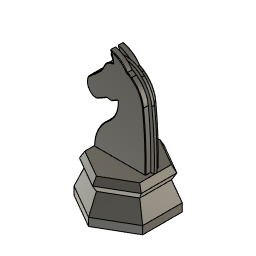
Knight Chess Piece (Autodesk Fusion 360 design; units mm, degrees)
Autodesk Fusion 360 part; units mm, degrees
sketch "Sketch2" plane through (0, 0, 0) normal (0, 0, 1) x (1, 0, 0)
  line L0 (0, 15) -> (-12.990381, 7.5)
  line L1 (-12.990381, 7.5) -> (-12.990381, -7.5)
  line L2 (-12.990381, -7.5) -> (0, -15)
  line L3 (0, -15) -> (12.990381, -7.5)
  line L4 (12.990381, -7.5) -> (12.990381, 7.5)
  line L5 (12.990381, 7.5) -> (0, 15)
  dimension "d4" = 15
  measures "d4" distance of L0.start origin
extrude "Extrude1" add sketch "Sketch2" along normal blind 3 contours L0 L1 L2 L3 L4 L5 picked at (4.330127, 2.5)
sketch "Sketch3" plane through (0, 0, 3) normal (0, 0, 1) x (-1, 0, 0)
  line L0 (-12.990381, -7.5) -> (0, -15)
  line L1 (0, -15) -> (12.990381, -7.5)
  line L2 (12.990381, -7.5) -> (12.990381, 7.5)
  line L3 (12.990381, 7.5) -> (0, 15)
  line L4 (0, 15) -> (-12.990381, 7.5)
  line L5 (-12.990381, 7.5) -> (-12.990381, -7.5)
  line L6 (0, -15) -> (12.990381, -7.5)
  line L7 (12.990381, -7.5) -> (12.990381, 7.5)
  line L8 (12.990381, 7.5) -> (0, 15)
  line L9 (0, 15) -> (-12.990381, 7.5)
  line L10 (-12.990381, 7.5) -> (-12.990381, -7.5)
  line L11 (-12.990381, -7.5) -> (0, -15)
  constraint coincident L0.end L1.start
ref_plane "WorkPlane1" through (0, 0, 10) normal (0, 0, 1) x (-1, 0, 0)
sketch "Sketch4" plane through (0, 0, 10) normal (0, 0, 1) x (1, 0, 0)
  line L0 (0, 12) -> (-10.392305, 6)
  line L1 (-10.392305, 6) -> (-10.392305, -6)
  line L2 (-10.392305, -6) -> (0, -12)
  line L3 (0, -12) -> (10.392305, -6)
  line L4 (10.392305, -6) -> (10.392305, 6)
  line L5 (10.392305, 6) -> (0, 12)
  dimension "d8" = 12
  measures "d8" distance of L0.start origin
loft "Loft1" add profiles "Sketch3", "Sketch4" section 1 contours L0 L1 L2 L3 L4 L5 L6 L7 L8 L9 L10 L11 picked at (-4.330127, -2.5) section 2 contours L0 L1 L2 L3 L4 L5 picked at (0, 0)
sketch "Sketch5" plane through (0, 0, 10) normal (0, 0, 1) x (-1, 0, 0)
  line L0 (-10.392305, -6) -> (0, -12)
  line L1 (0, -12) -> (10.392305, -6)
  line L2 (10.392305, -6) -> (10.392305, 6)
  line L3 (10.392305, 6) -> (0, 12)
  line L4 (0, 12) -> (-10.392305, 6)
  line L5 (-10.392305, 6) -> (-10.392305, -6)
  line L6 (0, -12) -> (10.392305, -6)
  line L7 (10.392305, -6) -> (10.392305, 6)
  line L8 (10.392305, 6) -> (0, 12)
  line L9 (0, 12) -> (-10.392305, 6)
  line L10 (-10.392305, 6) -> (-10.392305, -6)
  line L11 (-10.392305, -6) -> (0, -12)
  constraint coincident L0.end L1.start
ref_plane "WorkPlane2" through (0, 0, 12.5) normal (0, 0, 1) x (-1, 0, 0)
sketch "Sketch6" plane through (0, 0, 12.5) normal (0, 0, 1) x (1, 0, 0)
  line L0 (0, 13.5) -> (-11.691343, 6.75)
  line L1 (-11.691343, 6.75) -> (-11.691343, -6.75)
  line L2 (-11.691343, -6.75) -> (0, -13.5)
  line L3 (0, -13.5) -> (11.691343, -6.75)
  line L4 (11.691343, -6.75) -> (11.691343, 6.75)
  line L5 (11.691343, 6.75) -> (0, 13.5)
  line L6 (0, 15) -> (0, 12)
  constraint midpoint L0.start L6
ref_plane "WorkPlane3" through (0, 0, 15) normal (0, 0, 1) x (1, 0, 0)
sketch "Sketch7" plane through (0, 0, 15) normal (0, 0, 1) x (1, 0, 0)
  line L0 (0, 12) -> (-10.392305, 6)
  line L1 (-10.392305, 6) -> (-10.392305, -6)
  line L2 (-10.392305, -6) -> (0, -12)
  line L3 (0, -12) -> (10.392305, -6)
  line L4 (10.392305, -6) -> (10.392305, 6)
  line L5 (10.392305, 6) -> (0, 12)
  point P0 (0, 12)
  constraint coincident P0 L0.start
loft "Loft2" add profiles "Sketch5", "Sketch6" section 1 contours L0 L1 L2 L3 L4 L5 L6 L7 L8 L9 L10 L11 picked at (-3.464102, 2) section 2 contours L0 L1 L2 L3 L4 L5 picked at (3.897114, 2.25)
sketch "Sketch8" plane through (0, 0, 12.5) normal (0, 0, 1) x (-1, 0, 0)
  line L0 (-11.691343, -6.75) -> (0, -13.5)
  line L1 (0, -13.5) -> (11.691343, -6.75)
  line L2 (11.691343, -6.75) -> (11.691343, 6.75)
  line L3 (11.691343, 6.75) -> (0, 13.5)
  line L4 (0, 13.5) -> (-11.691343, 6.75)
  line L5 (-11.691343, 6.75) -> (-11.691343, -6.75)
  line L6 (0, -13.5) -> (11.691343, -6.75)
  line L7 (11.691343, -6.75) -> (11.691343, 6.75)
  line L8 (11.691343, 6.75) -> (0, 13.5)
  line L9 (0, 13.5) -> (-11.691343, 6.75)
  line L10 (-11.691343, 6.75) -> (-11.691343, -6.75)
  line L11 (-11.691343, -6.75) -> (0, -13.5)
  constraint coincident L0.end L1.start
loft "Loft3" add profiles "Sketch8", "Sketch7" section 1 contours L0 L1 L2 L3 L4 L5 L6 L7 L8 L9 L10 L11 picked at (-3.897114, -2.25) section 2 contours L0 L1 L2 L3 L4 L5 picked at (0, 0)
shell "Shell1" thickness 2 removed faces 1 at (4.330127, 2.5, 0)
sketch "Sketch10" plane through (0, 0, 0) normal (0, 1, 0) x (1, 0, 0)
  line L0 (-15, 0) -> (15, 0) construction
  line L1 (15, 0) -> (15, -50) construction
  line L2 (15, -50) -> (-15, -50) construction
  line L3 (-15, -50) -> (-15, 0) construction
  line L4 (0, 0) -> (0, -50.000001) construction
  arc A0 (-10.392305, -15) -> (-5.031411, -25.974647) centre (4.068204, -14.733001) ccw
  arc A1 (-1.45223, -34.282944) -> (-5.031411, -25.974647) centre (-11.152568, -33.536714) ccw
  line L5 (-1.45223, -34.282944) -> (-3.369432, -33.194671)
  arc A2 (-3.369432, -33.194671) -> (-5.5, -33.194671) centre (-4.434716, -35.071372) ccw
  line L6 (-5.5, -33.194671) -> (-9.003186, -31.206135)
  arc A3 (-9.003186, -31.206135) -> (-11, -31.206135) centre (-10.001593, -32.965019) ccw
  arc A4 (-11, -31.206135) -> (-12.660134, -36.669443) centre (-8.953188, -34.811985) ccw
  line L7 (-12.660134, -36.669443) -> (-8.504363, -40.327582)
  arc A5 (-6.723878, -42.918601) -> (-8.504363, -40.327582) centre (-12.7535, -45.154747) ccw
  arc A6 (-4.682649, -45.182039) -> (3.634445, -44.218793) centre (-1.386515, -37.253958) ccw
  arc A7 (3.634445, -44.218793) -> (8.13983, -36.485073) centre (-2.802633, -35.289588) ccw
  line L8 (10.392305, -15) -> (0, -15)
  arc A8 (8.13983, -36.485073) -> (9.030382, -15) centre (-150.571914, -19.145511) ccw
  line L9 (-10.392305, -15) -> (9.030382, -15)
  arc A9 (-6.723878, -42.918601) -> (-4.682649, -45.182039) centre (-2.858972, -41.485262) ccw
  point P0 (-10.392305, -15)
  dimension "d13" = 30
  dimension "d14" = 50
  dimension "d15" = 15
  constraint horizontal L0
  constraint vertical L1
  constraint horizontal L2
  constraint coincident L4.start origin
  constraint perpendicular L2 L4
  constraint tangent A0 A1
  constraint tangent L5 A2
  constraint parallel L5 L6
  constraint tangent L6 A3
  constraint tangent A3 A4
  constraint tangent L7 A5
  constraint tangent A6 A7
  constraint tangent A7 A8
  constraint tangent A5 A9
  measures "d13" distance of L0.start L0.end
  measures "d14" distance of L0.start L2.end
  measures "d15" distance of L3 L4
extrude "Extrude2" add sketch "Sketch10" along normal mid plane 5 contours A0 A1 L5 A2 L6 A3 A4 L7 A5 A6 A7 L8 A8 L9 A9 picked at (1.669067, -21.354104)
sketch "Sketch12" plane through (0, 0, 0) normal (0, 1, 0) x (1, 0, 0)
  line L0 (-10.392305, -15) -> (8.638266, -15.045559)
  line L1 (-12.660134, -36.669443) -> (-8.504363, -40.327582)
  arc A0 (-11, -31.206135) -> (-12.660134, -36.669443) centre (-8.953188, -34.811985) ccw
  arc A1 (-5.268961, -44.810581) -> (4.41457, -43.289947) centre (-1.520828, -37.085915) ccw
  arc A2 (-7.025416, -42.576626) -> (-8.504363, -40.327582) centre (-11.871086, -44.152295) ccw
  arc A3 (-10.392305, -15) -> (-5.031411, -25.974647) centre (4.068204, -14.733001) ccw
  arc A4 (-1.45223, -34.282944) -> (-5.031411, -25.974647) centre (-11.152568, -33.536714) ccw
  arc A5 (7.7476, -36.53168) -> (8.638266, -15.045559) centre (-150.964029, -19.19107) ccw
  arc A6 (-3.369432, -33.194671) -> (-5.5, -33.194671) centre (-4.434716, -35.071372) ccw
  arc A7 (-9.003186, -31.206135) -> (-11, -31.206135) centre (-10.001593, -32.965019) ccw
  arc A8 (4.41457, -43.289947) -> (7.7476, -36.53168) centre (-3.194854, -35.336122) ccw
  arc A9 (-7.025416, -42.576626) -> (-5.268961, -44.810581) centre (-3.105326, -41.301929) ccw
  line L2 (-1.45223, -34.282944) -> (-3.369432, -33.194671)
  line L3 (-5.5, -33.194671) -> (-9.003186, -31.206135)
  arc A10 (-6.03493, -46.389194) -> (5.627528, -44.557803) centre (-1.520828, -37.085915) ccw
  arc A11 (5.627528, -44.557803) -> (9.49185, -36.722254) centre (-3.194854, -35.336122) ccw
  arc A12 (9.49185, -36.722254) -> (10.392305, -15) centre (-150.964029, -19.19107) ccw
  line L4 (-6.03493, -46.389194) -> (-5.268961, -44.810581)
  line L5 (-10.392305, -15) -> (9.030382, -15)
  line L6 (8.638266, -15.045559) -> (8.637083, -15)
  line L7 (10.392305, -15) -> (8.637083, -15)
  point P0 (-10.392305, -15)
  point P1 (10.392305, -15)
  dimension "d18" = 1.75463
  constraint tangent A3 A4
  constraint tangent A6 L2
  constraint parallel L2 L3
  constraint tangent A7 L3
  constraint tangent A0 A7
  constraint tangent L1 A2
  constraint tangent A1 A8
  constraint tangent A5 A8
  constraint tangent A2 A9
  constraint tangent A5 L6
extrude "Extrude3" add sketch "Sketch12" along normal mid plane 1 contours A1 A5 A8 A10 A11 A12 L4 L5 L6 L7 picked at (9.370491, -19.823446)
sketch "Sketch14" plane through (0, -2.5, 0) normal (0, -1, 0) x (1, 0, 0)
  line L0 (-3.369432, 33.194671) -> (-1.45223, 34.282944)
  arc A0 (-5.031411, 25.974647) -> (-1.45223, 34.282944) centre (-11.152568, 33.536714) ccw
  arc A1 (-5.031411, 25.974647) -> (-10.392305, 15) centre (4.068204, 14.733001) ccw
  line L1 (-10.392305, 15) -> (9.030382, 15)
  arc A2 (9.030382, 15) -> (8.13983, 36.485073) centre (-150.571914, 19.145511) ccw
  arc A3 (8.13983, 36.485073) -> (3.634445, 44.218793) centre (-2.802633, 35.289588) ccw
  arc A4 (3.634445, 44.218793) -> (-4.682649, 45.182039) centre (-1.386515, 37.253958) ccw
  arc A5 (-4.682649, 45.182039) -> (-6.723878, 42.918601) centre (-2.858972, 41.485262) ccw
  arc A6 (-8.504363, 40.327582) -> (-6.723878, 42.918601) centre (-12.7535, 45.154747) ccw
  line L2 (-8.504363, 40.327582) -> (-12.660134, 36.669443)
  arc A7 (-12.660134, 36.669443) -> (-11, 31.206135) centre (-8.953188, 34.811985) ccw
  arc A8 (-11, 31.206135) -> (-9.003186, 31.206135) centre (-10.001593, 32.965019) ccw
  line L3 (-9.003186, 31.206135) -> (-5.5, 33.194671)
  arc A9 (-5.5, 33.194671) -> (-3.369432, 33.194671) centre (-4.434716, 35.071372) ccw
  arc A10 (3.634445, 44.218793) -> (-4.682649, 45.182039) centre (-1.386515, 37.253958) ccw
  arc A11 (-3.187309, 45.648963) -> (-4.3, 49.499999) centre (-12.407676, 45.071161) ccw
  arc A12 (2.02935, 45.131193) -> (-4.3, 49.499999) centre (-6.29726, 39.837194) ccw
extrude "Extrude4" add sketch "Sketch14" against normal blind 2 contours A4 A10 A11 A12 picked at (-2.441936, 47.140274)
mirror "Mirror1" about plane through (0, 0, 0) normal (0, 1, 0) of "Extrude4"
fillet "Fillet1" radius 0.2 32 edges at (-5.920145, -2.5, 44.24591) (-7.453352, -2.5, 41.512615) (-10.582248, -2.5, 38.498512) (-3.94565, -2.5, 45.449676) (8.947235, -2.5, 25.757546) (6.708661, -2.5, 40.830523) (2.856493, -2.5, 44.718262) (-12.920349, -2.5, 33.606485) (-10.001593, -2.5, 30.942523) (-7.251593, -2.5, 32.200403) (-4.434716, -2.5, 32.913401) (-2.410831, -2.5, 33.738808) (-2.21742, -2.5, 29.687488) (-8.927202, -2.5, 21.080995) (-3.532267, -2.5, 47.635558) (-0.692156, -2.5, 47.957641) (-3.532267, 2.5, 47.635558) (-0.692156, 2.5, 47.957641) (2.856493, 2.5, 44.718262) (6.708661, 2.5, 40.830523) (8.947235, 2.5, 25.757546) (-3.94565, 2.5, 45.449676) (-10.582248, 2.5, 38.498512) (-7.453352, 2.5, 41.512615) (-5.920145, 2.5, 44.24591) (-7.251593, 2.5, 32.200403) (-10.001593, 2.5, 30.942523) (-12.920349, 2.5, 33.606485) (-2.410831, 2.5, 33.738808) (-4.434716, 2.5, 32.913401) (-8.927202, 2.5, 21.080995) (-2.21742, 2.5, 29.687488)
